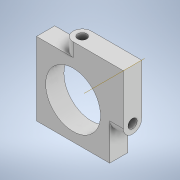
# Autodesk Inventor part: PivotHolder
Saved by Autodesk Inventor 2022.2 (Build 262287030, 287C)
## iProperties
Created: 2023-04-03
Part Number: PivotHolder
Material: Generic
Document SubType Name: Modeling
Designer: jak27277
Density: 1 g/cm^3
Appearance: Default
Author: jak27277
Autodesk Inventor part; units mm, degrees
note: some values were not read from the file. Chosen so that the rebuilt part matches the saved one: direction of "Hole2"; direction of "Hole3".
ref_plane "YZ Plane" through (0, 0, 0) normal (1, 0, 0) x (0, 1, 0)
ref_plane "XZ Plane" through (0, 0, 0) normal (0, 1, 0) x (-1, 0, 0)
ref_plane "XY Plane" through (0, 0, 0) normal (0, 0, 1) x (1, 0, 0)
sketch "Sketch2" plane through (0, 0, 0) normal (0, 1, 0) x (-1, 0, 0)
  line L0 (0, 0) -> (69.85, 0)
  line L1 (69.85, 0) -> (69.85, -25.4) construction
  line L2 (69.85, -25.4) -> (0, -25.4)
  line L3 (0, -25.4) -> (0, 0)
  arc A0 (69.85, -25.4) -> (69.85, 0) centre (69.85, -12.7) ccw
  dimension "d0" = 25.4
  dimension "d1" = 69.85
  constraints: 8 end point, 2 parallel, 2 point on circle, 1 centre point, 1 horizontal, 1 perpendicular, 1 tangent
  measures "d0" distance of L2.end L0.start
  measures "d1" distance of L1.end L2.end
extrude "Extrusion1" add sketch "Sketch2" along normal blind 19.05
ref_plane "Work Plane1" through (0, 19.05, 0) normal (0.7071068, -0.7071068, 0) x (0, 0, -1)
mirror "Mirror1" about plane through (0, 19.05, 0) normal (0.7071068, -0.7071068, 0) of "Extrusion1"
sketch "Sketch3" plane through (-69.85, 19.05, 0) normal (0, 0, 1) x (1, 0, 0)
  line L0 (50.8, -69.85) -> (50.8, -19.05) projected
  line L1 (-50.8, -120.65) -> (50.8, -120.65)
  line L2 (50.8, -120.65) -> (50.8, -19.05)
  line L3 (50.8, -19.05) -> (-50.8, -19.05)
  line L4 (-50.8, -19.05) -> (-50.8, -120.65)
  line L5 (-50.8, -120.65) -> (50.8, -19.05) construction
  line L6 (50.8, -120.65) -> (-50.8, -19.05) construction
  point P0 (0, -69.85)
  point P1 (0, -69.85)
  dimension "d6" = 101.6
  constraints: 12 end point, 2 midpoint, 2 parallel, 2 perpendicular, 1 coincident, 1 horizontal
  measures "d6" distance of L0.end L3.end
extrude "Extrusion2" add sketch "Sketch3" against normal up to surface (25.4 mm away)
hole "Hole1" at (-69.85, -50.8, 0) direction (0, 0, -1) diameter 76.2 end through all
sketch "Sketch4" plane through (0, 19.05, 0) normal (1, 0, 0) x (0, 0, -1)
  arc A0 (0, -69.85) -> (25.4, -69.85) centre (12.7, -69.85) ccw projected
  point P0 (0, -19.05)
  constraints: 2 coincident
hole "Hole2" at (0, -50.8, -12.7) direction (-1, 0, 0) diameter 12.7 end up to surface
sketch "Sketch5" plane through (0, 19.05, 0) normal (0, 1, 0) x (1, 0, 0)
  arc A0 (-69.85, 25.4) -> (-69.85, 0) centre (-69.85, 12.7) ccw projected
  point P0 (0, 0)
  constraints: 1 coincident
hole "Hole3" at (-69.85, 19.05, -12.7) direction (0, -1, 0) diameter 12.7 end up to surface
body "Solid1"
